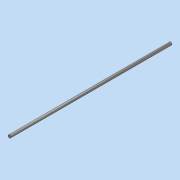
# Autodesk Inventor part: PistonSupportRod
Saved by Autodesk Inventor 2017.3 (Build 213256000, 256)
## iProperties
Created: 2016-12-01
Part Number: PistonSupportRod
Material: Steel, Carbon
Document SubType Name: Modeling
Designer: techn
Density: 7.85 g/cm^3
Appearance: Semi-Polished
Author: techn
Autodesk Inventor part; units mm, degrees
ref_plane "YZ Plane" through (0, 0, 0) normal (1, 0, 0) x (0, 1, 0)
ref_plane "XZ Plane" through (0, 0, 0) normal (0, 1, 0) x (-1, 0, 0)
ref_plane "XY Plane" through (0, 0, 0) normal (0, 0, 1) x (1, 0, 0)
sketch "Sketch1" plane through (0, 0, 0) normal (0, 0, 1) x (1, 0, 0)
  circle A0 centre (0, 0) radius 1.5875
  dimension "d0" = 3.175
  constraints: 1 centre point, 1 coincident
  measures "d0" diameter of A0
extrude "Extrusion1" add sketch "Sketch1" along normal blind 168.5036
body "Solid1"
